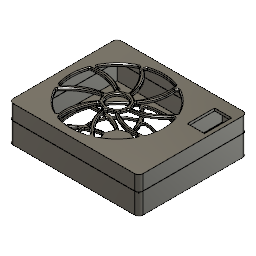
120mm_Solder_Fume_Extractor (Autodesk Fusion 360 design; units mm, degrees)
Autodesk Fusion 360 part; units mm, degrees
sketch "Skizze1" plane through (0, 0, 0) normal (0, 1, 0) x (1, 0, 0)
  circle A0 centre (-52.5, 52.5) radius 2.5
  line L0 (1.75, 0) -> (22.5, 0)
  line L1 (0, -1.75) -> (0, -22.5)
  circle A1 centre (-52.5, -52.5) radius 2.5
  circle A2 centre (52.5, 52.5) radius 2.5
  circle A3 centre (52.5, -52.5) radius 2.5
  line L2 (65, 65) -> (-65, 65)
  line L3 (-65, 65) -> (-65, -65)
  line L4 (-65, -65) -> (65, -65)
  line L5 (65, -65) -> (65, 65)
  line L6 (65, 65) -> (-65, -65) construction
  line L7 (-65, 65) -> (65, -65) construction
  circle A4 centre (0, 0) radius 55
  dimension "d1" = 5
  dimension "d2" = 5
  dimension "d3" = 5
  dimension "d4" = 5
  dimension "d5" = 105
  dimension "d6" = 105
  dimension "d7" = 130
  dimension "d8" = 130
  dimension "d9" = 110
  constraint symmetric A0 L1 A2
  constraint symmetric A0 L0 A1
  constraint symmetric L0 A2 A3
  constraint symmetric L1 A1 A3
  constraint perpendicular L2 L3
  constraint parallel L2 L4
  constraint parallel L3 L5
  constraint horizontal L2
  constraint coincident L6 A4.centre
  constraint coincident L7 A4.centre
  constraint coincident A4.centre origin
  measures "d1" diameter of A0
  measures "d2" diameter of A1
  measures "d3" diameter of A2
  measures "d4" diameter of A3
  measures "d5" vertical distance of A0.centre A1.centre
  measures "d6" horizontal distance of A0.centre A2.centre
  measures "d7" distance of L2.end L3.end
  measures "d8" distance of L3.end L4.end
  measures "d9" diameter of A4
extrude "Extrusion1" add sketch "Skizze1" along normal blind 3 makes body 1
sketch "Skizze2" plane through (0, 0, 0) normal (0, 1, 0) x (1, 0, 0)
  circle A0 centre (0, 0) radius 15
  circle A1 centre (0, 0) radius 55
  arc A2 (0, 0) -> (-18.8111, -51.6831) centre (39.1969, -43.5314) ccw
  arc A3 (0, 0) -> (-21.9924, -50.4117) centre (22.9762, -40.0265) ccw
  dimension "d12" = 30
  constraint coincident A0.centre A1.centre
  measures "d12" diameter of A0
extrude "Extrusion2" add sketch "Skizze2" along normal blind 3 separate body contours A0 A2 A3 | A0 A1 A2 A3 picked at (-8.6621, -7.7901) picked at (-19.3508, -31.0789) makes body 2
sketch "Skizze3" plane through (0, 3, 0) normal (0, 1, 0) x (-1, 0, 0)
  circle A0 centre (-52.5, 52.5) radius 2.5
  circle A1 centre (52.5, -52.5) radius 2.5
  circle A2 centre (-52.5, -52.5) radius 2.5
  circle A3 centre (52.5, 52.5) radius 2.5
  line L0 (-65, 65) -> (-65, -65)
  line L1 (-65, -65) -> (65, -65)
  line L2 (65, -65) -> (65, 65)
  line L3 (65, 65) -> (-65, 65)
  line L4 (65, -65) -> (61, -65)
  line L5 (61, -65) -> (61, 65)
  line L6 (61, 65) -> (65, 65)
  line L7 (65, 65) -> (65, -65)
  line L8 (65, 65) -> (-65, 65)
  line L9 (-65, 65) -> (-65, 61)
  line L10 (-65, 61) -> (65, 61)
  line L11 (65, 61) -> (65, 65)
  line L12 (-65, 65) -> (-61, 65)
  line L13 (-61, 65) -> (-61, -65)
  line L14 (-61, -65) -> (-65, -65)
  line L15 (-65, -65) -> (-65, 65)
  line L16 (-65, -65) -> (65, -65)
  line L17 (65, -65) -> (65, -61)
  line L18 (65, -61) -> (-65, -61)
  line L19 (-65, -61) -> (-65, -65)
  circle A4 centre (0, 0) radius 55
  dimension "d15" = 4
  dimension "d16" = 4
  dimension "d17" = 4
  dimension "d18" = 4
  constraint horizontal L4
  constraint vertical L5
  constraint horizontal L6
  constraint vertical L7
  constraint coincident L1.end L2.start
  constraint horizontal L8
  constraint vertical L9
  constraint horizontal L10
  constraint vertical L11
  constraint horizontal L12
  constraint vertical L13
  constraint horizontal L14
  constraint vertical L15
  constraint horizontal L16
  constraint vertical L17
  constraint horizontal L18
  constraint vertical L19
  constraint coincident L2 L17.end
  measures "d15" distance of L1.end L4.end
  measures "d16" distance of L2.end L10.end
  measures "d17" distance of L0.start L12.end
  measures "d18" distance of L0.end L18.end
extrude "Extrusion3" add sketch "Skizze3" along normal blind 20 contours L0 L3 L8 L9 L10 L12 L13 L15 | L0 L10 L13 L15 L18 | L3 L5 L8 L10 L13 | L0 L1 L13 L14 L15 L16 L18 L19 | L2 L3 L5 L6 L7 L8 L10 L11 | L1 L5 L13 L16 L18 | L2 L5 L7 L10 L18 | L1 L2 L4 L5 L7 L16 L17 L18 bodies 1
sketch "Skizze4" plane through (0, 0, 0) normal (0, 1, 0) x (1, 0, 0)
  line L0 (65, -65) -> (91, -65)
  line L1 (91, -65) -> (91, 65)
  line L2 (91, 65) -> (65, 65)
  line L3 (65, 65) -> (65, -65)
  point P0 (65, -65)
  dimension "d21" = 26
  constraint horizontal L0
  constraint vertical L1
  constraint horizontal L2
  constraint vertical L3
  constraint coincident P0 L0.start
  measures "d21" distance of P0 L0.end
extrude "Extrusion4" add sketch "Skizze4" along normal blind 3 bodies 1
sketch "Skizze5" plane through (0, 3, 0) normal (0, 1, 0) x (-1, 0, 0)
  line L0 (-65, -65) -> (-65, 65)
  line L1 (-65, 65) -> (-91, 65)
  line L2 (-91, 65) -> (-91, -65)
  line L3 (-91, -65) -> (-65, -65)
  line L4 (-91, -65) -> (-65, -65)
  line L5 (-65, -65) -> (-65, -61)
  line L6 (-65, -61) -> (-91, -61)
  line L7 (-91, -61) -> (-91, -65)
  line L8 (-91, 65) -> (-87, 65)
  line L9 (-87, 65) -> (-87, -65)
  line L10 (-87, -65) -> (-91, -65)
  line L11 (-91, -65) -> (-91, 65)
  line L12 (-91, 65) -> (-65, 65)
  line L13 (-65, 65) -> (-65, 61)
  line L14 (-65, 61) -> (-91, 61)
  line L15 (-91, 61) -> (-91, 65)
  dimension "d24" = 4
  dimension "d25" = 4
  dimension "d26" = 4
  constraint horizontal L4
  constraint vertical L5
  constraint horizontal L6
  constraint vertical L7
  constraint coincident L2.end L3.start
  constraint horizontal L8
  constraint vertical L9
  constraint horizontal L10
  constraint vertical L11
  constraint coincident L1.end L2.start
  constraint horizontal L12
  constraint vertical L13
  constraint horizontal L14
  constraint vertical L15
  measures "d24" distance of L2.end L6.end
  measures "d25" distance of L1.end L8.end
  measures "d26" distance of L1.end L14.end
extrude "Extrusion5" add sketch "Skizze5" along normal blind 20 contours L0 L3 L4 L5 L6 L9 | L2 L3 L4 L6 L7 L9 L10 L11 | L0 L1 L9 L12 L13 L14 | L2 L6 L9 L11 L14 | L1 L2 L8 L9 L11 L12 L14 L15 bodies 1
sketch "Skizze6" plane through (0, 0, -61) normal (0, 0, 1) x (1, 0, 0)
  line L0 (65, 3) -> (87, 3)
  line L1 (87, 3) -> (87, 23)
  line L2 (87, 23) -> (65, 23)
  line L3 (65, 23) -> (65, 3)
  line L4 (67, 23) -> (85, 23)
  line L5 (85, 23) -> (85, 21)
  line L6 (85, 21) -> (67, 21)
  line L7 (67, 21) -> (67, 23)
  line L8 (71.5, 21) -> (80.5, 21)
  line L9 (80.5, 21) -> (80.5, 17)
  line L10 (80.5, 17) -> (71.5, 17)
  line L11 (71.5, 17) -> (71.5, 21)
  dimension "d29" = 18
  dimension "d31" = 9
  dimension "d32" = 4
  dimension "d33" = 4.5
  constraint horizontal L4
  constraint vertical L5
  constraint horizontal L6
  constraint vertical L7
  constraint coincident L2 L4.start
  constraint horizontal L8
  constraint vertical L9
  constraint horizontal L10
  constraint vertical L11
  constraint coincident L6 L8.start
  measures "d29" distance of L4.start L4.end
  measures "d31" distance of L8.start L8.end
  measures "d32" distance of L8.start L10.end
  measures "d33" distance of L7 L11
extrude "Extrusion6" cut sketch "Skizze6" against normal blind 4 contours L2 L4 L5 L6 L7 L8 | L6 L8 L9 L10 L11 bodies 1
sketch "Skizze7" plane through (0, 23, 0) normal (0, 1, 0) x (-1, 0, 0)
  line L0 (-61, -61) -> (-61, 61)
  line L1 (-61, 61) -> (61, 61)
  line L2 (61, 61) -> (61, -61)
  line L3 (61, -61) -> (-61, -61)
  line L4 (-65, 61) -> (-65, -61)
  line L5 (-67, -65) -> (65, -65)
  line L6 (65, -65) -> (65, 65)
  line L7 (65, 65) -> (-91, 65)
  line L8 (65, 65) -> (63, 65)
  line L9 (63, -65) -> (65, -65)
  line L10 (65, -65) -> (65, 65)
  line L11 (65, 65) -> (-65, 65)
  line L12 (-65, 65) -> (-65, 63.2)
  line L13 (-65, 63.2) -> (65, 63.2)
  line L14 (65, 63.2) -> (65, 65)
  line L15 (65, -65) -> (-65, -65)
  line L16 (-65, -65) -> (-65, -63)
  line L17 (65, -63) -> (65, -65)
  line L18 (65, 65) -> (63.2, 65)
  line L19 (63.2, 65) -> (63.2, -65)
  line L20 (63.2, -65) -> (65, -65)
  line L21 (65, -65) -> (65, 65)
  line L22 (65, -65) -> (-65, -65)
  line L23 (-65, -65) -> (-65, -63.2)
  line L24 (-65, -63.2) -> (65, -63.2)
  line L25 (65, -63.2) -> (65, -65)
  line L26 (-67, -61) -> (-67, -65)
  line L27 (-91, 65) -> (-91, -65)
  line L28 (-91, -65) -> (-85, -65)
  line L29 (-85, -65) -> (-85, -61)
  line L30 (-85, -61) -> (-87, -61)
  line L31 (-87, -61) -> (-87, 61)
  line L32 (-87, 61) -> (-65, 61)
  line L33 (-65, -61) -> (-67, -61)
  dimension "d36" = 2
  dimension "d37" = 1.8
  dimension "d46" = 1.8
  dimension "d47" = 1.8
  constraint horizontal L8
  constraint horizontal L9
  constraint vertical L10
  constraint coincident L6.end L7.start
  constraint horizontal L11
  constraint vertical L12
  constraint horizontal L13
  constraint vertical L14
  constraint horizontal L15
  constraint vertical L16
  constraint coincident L5.end L6.start
  constraint horizontal L18
  constraint vertical L19
  constraint horizontal L20
  constraint vertical L21
  constraint horizontal L22
  constraint vertical L23
  constraint horizontal L24
  constraint vertical L25
  measures "d36" distance of L6.end L8.end
  measures "d37" distance of L6.end L13.end
  measures "d46" distance of L6.end L18.end
  measures "d47" distance of L5.end L24.end
extrude "Extrusion7" add sketch "Skizze7" along normal blind 2 contours L5 L9 L15 L16 L19 L22 L23 L24 | L5 L6 L9 L10 L15 L17 L19 L20 L21 L22 L24 L25 | L6 L10 L13 L17 L19 L21 L24 | L6 L7 L8 L10 L11 L13 L14 L18 L19 L21 | L7 L8 L11 L12 L13 L19 bodies 1
sketch "Skizze8" plane through (0, 23, 0) normal (0, 1, 0) x (-1, 0, 0)
  line L0 (-85, -65) -> (-85, -61)
  line L1 (-85, -61) -> (-87, -61)
  line L2 (-87, -61) -> (-87, 61)
  line L3 (-87, 61) -> (-65, 61)
  line L4 (-65, 65) -> (-91, 65)
  line L5 (-91, 65) -> (-91, -65)
  line L6 (-91, -65) -> (-85, -65)
  line L7 (-85, -65) -> (-91, -65)
  line L8 (-91, -65) -> (-91, -63.2)
  line L9 (-91, -63.2) -> (-85, -63.2)
  line L10 (-85, -63.2) -> (-85, -65)
  line L11 (-91, -65) -> (-89.2, -65)
  line L12 (-89.2, -65) -> (-89.2, 65)
  line L13 (-89.2, 65) -> (-91, 65)
  line L14 (-91, 65) -> (-91, -65)
  line L15 (-91, 65) -> (-65, 65)
  line L16 (-65, 65) -> (-65, 63.2)
  line L17 (-65, 63.2) -> (-91, 63.2)
  line L18 (-91, 63.2) -> (-91, 65)
  line L19 (-65, -65) -> (-67, -65)
  line L20 (-67, -65) -> (-67, -63.2)
  line L21 (-67, -63.2) -> (-65, -63.2)
  line L22 (-65, -63.2) -> (-65, -65)
  line L23 (-61, -61) -> (-61, 61)
  line L24 (-61, 61) -> (61, 61)
  line L25 (61, 61) -> (61, -61)
  line L26 (61, -61) -> (-61, -61)
  line L27 (-65, -65) -> (-65, -63.2)
  line L28 (-65, -63.2) -> (63.2, -63.2)
  line L29 (63.2, -63.2) -> (63.2, 63.2)
  line L30 (63.2, 63.2) -> (-65, 63.2)
  line L31 (-65, 63.2) -> (-65, 65)
  line L32 (-65, 61) -> (-65, -61)
  line L33 (-65, -61) -> (-67, -61)
  line L34 (-67, -61) -> (-67, -65)
  line L35 (-67, -65) -> (-65, -65)
  point P0 (-91, -65)
  point P1 (-67, -65)
  point P2 (-85, -65)
  point P3 (-65, -65)
  dimension "d40" = 1.8
  dimension "d41" = 1.8
  dimension "d42" = 1.8
  dimension "d43" = 1.8
  constraint horizontal L7
  constraint vertical L8
  constraint horizontal L9
  constraint vertical L10
  constraint coincident P2 L0.start
  constraint horizontal L11
  constraint vertical L12
  constraint horizontal L13
  constraint vertical L14
  constraint coincident P0 L5.end
  constraint horizontal L15
  constraint vertical L16
  constraint horizontal L17
  constraint vertical L18
  constraint horizontal L19
  constraint vertical L20
  constraint horizontal L21
  constraint vertical L22
  measures "d40" distance of P2 L9.end
  measures "d41" distance of P0 L11.end
  measures "d42" distance of L4.end L17.end
  measures "d43" distance of P3 L21.end
extrude "Extrusion8" add sketch "Skizze8" along normal blind 2 contours L0 L6 L7 L9 L10 L12 | L5 L6 L7 L8 L9 L11 L12 L14 | L5 L9 L12 L14 L17 | L4 L5 L12 L13 L14 L15 L17 L18 | L4 L12 L15 L16 L17 L31 | L19 L20 L21 L22 L27 L34 L35 bodies 1
ref_plane "Arbeitsebene2" through (13, 25.2, 0) normal (0, 1, 0) x (0, 0, 1)
sketch "Skizze29" plane through (13, 25.2, 0) normal (0, 1, 0) x (1, 0, 0)
  line L0 (-78, -65) -> (78, -65)
  line L1 (78, -65) -> (78, 65)
  line L2 (78, 65) -> (72, 65)
  line L3 (72, 65) -> (72, 63.2)
  line L4 (72, 63.2) -> (76.2, 63.2)
  line L5 (76.2, 63.2) -> (76.2, -63.2)
  line L6 (76.2, -63.2) -> (-76.2, -63.2)
  line L7 (-76.2, -63.2) -> (-76.2, 63.2)
  line L8 (-76.2, 63.2) -> (54, 63.2)
  line L9 (54, 63.2) -> (54, 65)
  line L10 (54, 65) -> (-78, 65)
  line L11 (-78, 65) -> (-78, -65)
  line L12 (76.2, 63.2) -> (72, 63.2)
  line L13 (72, 63.2) -> (72, 61)
  line L14 (72, 61) -> (74, 61)
  line L15 (74, 61) -> (74, -61)
  line L16 (74, -61) -> (52, -61)
  line L17 (52, -61) -> (52, 61)
  line L18 (52, 61) -> (54, 61)
  line L19 (54, 61) -> (54, 63.2)
  line L20 (54, 63.2) -> (-76.2, 63.2)
  line L21 (-76.2, 63.2) -> (-76.2, -63.2)
  line L22 (-76.2, -63.2) -> (76.2, -63.2)
  line L23 (76.2, -63.2) -> (76.2, 63.2)
  line L24 (48, 61) -> (48, -61)
  line L25 (48, -61) -> (-74, -61)
  line L26 (-74, -61) -> (-74, 61)
  line L27 (-74, 61) -> (48, 61)
  line L28 (54, 61) -> (58.5, 61)
  line L29 (58.5, 61) -> (58.5, 65)
  line L30 (58.5, 65) -> (54, 65)
  line L31 (54, 65) -> (54, 61)
  line L32 (58.5, 61) -> (67.5, 61)
  line L33 (67.5, 61) -> (67.5, 65)
  line L34 (67.5, 65) -> (58.5, 65)
  line L35 (58.5, 65) -> (58.5, 61)
  line L36 (67.5, 61) -> (72, 61)
  line L37 (72, 61) -> (72, 65)
  line L38 (72, 65) -> (67.5, 65)
  line L39 (67.5, 65) -> (67.5, 61)
extrude "Extrusion28" add sketch "Skizze29" along normal blind 15 separate body contours L0 L1 L2 L3 L4 L5 L6 L7 L8 L9 L10 L11 L12 L20 L21 L22 L23 L31 L37 | L9 L19 L28 L29 L30 L31 L35 | L3 L13 L33 L36 L37 L38 L39 | L4 L5 L6 L7 L8 L12 L13 L14 L15 L16 L17 L18 L19 L20 L21 L22 L23 L31 L37 | L29 L32 L33 L34 L35 L39 makes body 3
sketch "Skizze30" plane through (0, 40.2, 0) normal (0, 1, 0) x (-1, 0, 0)
  line L0 (-65, -61) -> (-87, -61)
  line L1 (-87, -61) -> (-87, 61)
  line L2 (-87, 61) -> (-65, 61)
  line L3 (-65, 61) -> (-65, -61)
  line L4 (61, 61) -> (61, -61)
  line L5 (61, -61) -> (-61, -61)
  line L6 (-61, -61) -> (-61, 61)
  line L7 (-61, 61) -> (61, 61)
  line L8 (-91, -65) -> (65, -65)
  line L9 (65, -65) -> (65, 65)
  line L10 (65, 65) -> (-91, 65)
  line L11 (-91, 65) -> (-91, -65)
  line L12 (-87, -61) -> (-65, -61)
  line L13 (-65, -61) -> (-65, 61)
  line L14 (-65, 61) -> (-87, 61)
  line L15 (-87, 61) -> (-87, -61)
  line L16 (61, -61) -> (61, 61)
  line L17 (61, 61) -> (-61, 61)
  line L18 (-61, 61) -> (-61, -61)
  line L19 (-61, -61) -> (61, -61)
  line L20 (65, -65) -> (-91, -65)
  line L21 (-91, -65) -> (-91, 65)
  line L22 (-91, 65) -> (65, 65)
  line L23 (65, 65) -> (65, -65)
  line L24 (-61, -61) -> (61, -61)
  line L25 (61, -61) -> (61, 61)
  line L26 (61, 61) -> (-61, 61)
  line L27 (-61, 61) -> (-61, -61)
  circle A0 centre (-52.5, 52.5) radius 2.5
  circle A1 centre (52.5, -52.5) radius 2.5
  circle A2 centre (-52.5, -52.5) radius 2.5
  circle A3 centre (52.5, 52.5) radius 2.5
  circle A4 centre (0, 0) radius 55
extrude "Extrusion29" add sketch "Skizze30" along normal blind 3 contours L0 L1 L2 L3 L12 L13 L14 L15 | L4 L5 L6 L7 L16 L17 L18 L19 L24 L25 L26 L27 | L8 L9 L10 L11 L20 L21 L22 L23 | A4 bodies 3
sketch "Skizze31" plane through (0, 25.2, 0) normal (0, -1, 0) x (1, 0, 0)
  line L0 (87, -61) -> (65, -61)
  line L1 (65, -61) -> (65, 61)
  line L2 (65, 61) -> (87, 61)
  line L3 (87, 61) -> (87, -61)
  line L4 (-61, -61) -> (-61, 61)
  line L5 (-61, 61) -> (61, 61)
  line L6 (61, 61) -> (61, -61)
  line L7 (61, -61) -> (-61, -61)
  line L8 (-65, -65) -> (91, -65)
  line L9 (91, -65) -> (91, 65)
  line L10 (91, 65) -> (-65, 65)
  line L11 (-65, 65) -> (-65, -65)
  line L12 (-65, 61.0488) -> (91, 61.0488)
  line L13 (91, 61.0488) -> (91, 62.8488)
  line L14 (91, 62.8488) -> (-65, 62.8488)
  line L15 (-65, 62.8488) -> (-65, 61.0488)
  line L16 (87, 62.8488) -> (88.8, 62.8488)
  line L17 (88.8, 62.8488) -> (88.8, -65)
  line L18 (88.8, -65) -> (87, -65)
  line L19 (87, -65) -> (87, 62.8488)
  line L20 (88.8, -61) -> (-65, -61)
  line L21 (-65, -61) -> (-65, -62.8)
  line L22 (-65, -62.8) -> (88.8, -62.8)
  line L23 (88.8, -62.8) -> (88.8, -61)
  line L24 (-61, -62.8) -> (-62.8, -62.8)
  line L25 (-62.8, -62.8) -> (-62.8, 65)
  line L26 (-62.8, 65) -> (-61, 65)
  line L27 (-61, 65) -> (-61, -62.8)
  line L28 (61, 61) -> (65, 61)
  line L29 (65, 61) -> (65, -61)
  line L30 (65, -61) -> (61, -61)
  line L31 (61, -61) -> (61, 61)
  dimension "d160" = 1.8
  dimension "d161" = 1.8
  dimension "d162" = 1.8
  dimension "d163" = 1.8
  constraint horizontal L12
  constraint vertical L13
  constraint horizontal L14
  constraint vertical L15
  constraint coincident L11 L12.start
  constraint horizontal L16
  constraint vertical L17
  constraint horizontal L18
  constraint vertical L19
  constraint coincident L14 L16.start
  constraint horizontal L20
  constraint vertical L21
  constraint horizontal L22
  constraint vertical L23
  constraint coincident L17 L20.start
  constraint horizontal L24
  constraint vertical L25
  constraint horizontal L26
  constraint vertical L27
  constraint coincident L22 L24.start
  constraint horizontal L28
  constraint vertical L29
  constraint horizontal L30
  constraint vertical L31
  constraint coincident L0.end L1.start
  constraint coincident L5.end L6.start
  measures "d160" distance of L12.start L14.end
  measures "d161" distance of L16.start L16.end
  measures "d162" distance of L20.start L22.end
  measures "d163" distance of L24.start L24.end
extrude "Extrusion30" add sketch "Skizze31" along normal blind 2 contours L0 L7 L19 L20 L22 L27 L30 | L17 L19 L20 L22 L23 | L3 L12 L17 L19 L20 | L1 L6 L20 L28 L29 L30 L31 | L12 L14 L16 L17 L19 | L12 L14 L19 L27 | L20 L22 L24 L25 L27 | L4 L12 L20 L25 L27 | L12 L14 L25 L27 bodies 3
sketch "Skizze32" plane through (0, 0, -62.8) normal (0, 0, -1) x (-1, 0, 0)
  line L0 (62.8, 25.2) -> (-88.8, 25.2)
  line L1 (-88.8, 25.2) -> (-88.8, 23.2)
  line L2 (-88.8, 23.2) -> (62.8, 23.2)
  line L3 (62.8, 23.2) -> (62.8, 25.2)
  line L4 (-84.8, 23.2) -> (-67.2274, 23.2)
  line L5 (-67.2274, 23.2) -> (-67.2274, 25.2)
  line L6 (-67.2274, 25.2) -> (-84.8, 25.2)
  line L7 (-84.8, 25.2) -> (-84.8, 23.2)
  line L8 (-67, 25) -> (-67, 21)
  line L9 (-85, 21) -> (-85, 25)
  dimension "d166" = 0.2274
  dimension "d167" = 0.2
  constraint horizontal L4
  constraint vertical L5
  constraint horizontal L6
  constraint vertical L7
  constraint coincident L0 L5.end
  constraint coincident L2 L4.start
  measures "d166" distance of L5 L8
  measures "d167" distance of L7 L9
extrude "Extrusion31" add sketch "Skizze32" along normal blind 2.2 contours L0 L2 L4 L5 L6 L7 bodies 3
extrude "Extrusion32" add 1 faces at (77.5, 17, -63.6667) along direction (0, 1, 0) blind 0.5 on bodies 1 bodies 1
extrude "Extrusion33" add 2 faces at (83.5, 21, -62.3333) (70, 21, -62.3333) along direction (0, 1, 0) blind 0.5 on bodies 1 bodies 1
sketch "Skizze33" plane through (0, 40.2, 0) normal (0, -1, 0) x (1, 0, 0)
  line L0 (65, 61) -> (65, -61)
  line L1 (65, -61) -> (87, -61)
  line L2 (87, -61) -> (87, 61)
  line L3 (87, 61) -> (65, 61)
  line L4 (65.75, -51) -> (86.25, -51)
  line L5 (86.25, -51) -> (86.25, -18.5)
  line L6 (86.25, -18.5) -> (65.75, -18.5)
  line L7 (65.75, -18.5) -> (65.75, -51)
  dimension "d174" = 20.5
  dimension "d175" = 32.5
  dimension "d176" = 0.75
  dimension "d177" = 10
  constraint horizontal L4
  constraint vertical L5
  constraint horizontal L6
  constraint vertical L7
  measures "d174" distance of L4.start L4.end
  measures "d175" distance of L4.start L6.end
  measures "d176" distance of L0 L7
  measures "d177" distance of L1 L4
extrude "Extrusion34" cut sketch "Skizze33" against normal blind 3 contours L4 L5 L6 L7 bodies 3
fillet "Abrundung33" radius 5 8 edges at (91, 12.5, -65) (91, 12.5, 65) (-65, 12.5, 65) (-65, 12.5, -65) (91, 34.2, -65) (91, 34.2, 65) (-65, 34.2, 65) (-65, 34.2, -65) on bodies 1 3
sketch "Skizze35" plane through (0, 43.2, 0) normal (0, 1, 0) x (-1, 0, 0)
  line L0 (-65.75, -51) -> (-86.25, -51)
  line L1 (-86.25, -51) -> (-86.25, -18.5)
  line L2 (-86.25, -18.5) -> (-65.75, -18.5)
  line L3 (-65.75, -18.5) -> (-65.75, -51)
  circle A0 centre (-52.5, 52.5) radius 2.5
  circle A1 centre (52.5, 52.5) radius 2.5
  circle A2 centre (-52.5, -52.5) radius 2.5
  circle A3 centre (52.5, -52.5) radius 2.5
  arc A4 (60, -65) -> (65, -60) centre (60, -60) ccw
  line L4 (65, -60) -> (65, 60)
  arc A5 (65, 60) -> (60, 65) centre (60, 60) ccw
  line L5 (60, 65) -> (-86, 65)
  arc A6 (-86, 65) -> (-91, 60) centre (-86, 60) ccw
  line L6 (-91, 60) -> (-91, -60)
  arc A7 (-91, -60) -> (-86, -65) centre (-86, -60) ccw
  line L7 (-86, -65) -> (60, -65)
  circle A8 centre (52.5, -52.5) radius 2.5
  circle A9 centre (52.5, 52.5) radius 2.5
  circle A10 centre (-52.5, 52.5) radius 2.5
  circle A11 centre (-52.5, -52.5) radius 2.5
extrude "Extrusion36" add sketch "Skizze35" against normal blind 3 contours A0 A10 | A1 A9 | A2 A11 | A3 A8 bodies 3
sketch "Skizze36" plane through (61, 0, 0) normal (-1, 0, 0) x (0, 0, 1)
  line L0 (-61, 3) -> (61, 3)
  line L1 (61, 3) -> (61, 23)
  line L2 (61, 23) -> (-61, 23)
  line L3 (-61, 23) -> (-61, 3)
  circle A0 centre (-35, 9) radius 2
  dimension "d185" = 4
  measures "d185" diameter of A0
extrude "Extrusion37" cut sketch "Skizze36" against normal blind 4 contours A0 bodies 1
sketch "Skizze38" plane through (0, 40.2, 0) normal (0, -1, 0) x (1, 0, 0)
  line L0 (61, 61) -> (-61, 61)
  line L1 (-61, 61) -> (-61, -61)
  line L2 (-61, -61) -> (61, -61)
  line L3 (61, -61) -> (61, 61)
  line L4 (-61, -61) -> (-61, -36)
  line L5 (-61, -61) -> (-36, -61)
  line L6 (-36, -61) -> (-61, -36)
  circle A0 centre (-52.5, -52.5) radius 2.25
  dimension "d194" = 4.5
  constraint coincident L1.end L2.start
  constraint coincident L1 L4.end
  constraint perpendicular L2 L4
  constraint coincident L2 L5.end
  measures "d194" diameter of A0
extrude "Extrusion39" add sketch "Skizze38" along normal blind 8 separate body contours L1 L2 L4 L5 L6 makes body 4
sketch "Skizze39" plane through (0, 40.2, 0) normal (0, 1, 0) x (-1, 0, 0)
  circle A0 centre (52.5, -52.5) radius 2.25
  line L0 (36, -61) -> (61, -61)
  line L1 (61, -61) -> (61, -36)
  line L2 (61, -36) -> (36, -61)
  line L3 (49.5606, -55.4394) -> (53.5759, -56.5153)
  line L4 (53.5759, -56.5153) -> (56.5153, -53.5759)
  line L5 (56.5153, -53.5759) -> (55.4394, -49.5606)
  line L6 (55.4394, -49.5606) -> (51.4241, -48.4847)
  line L7 (51.4241, -48.4847) -> (48.4847, -51.4241)
  line L8 (48.4847, -51.4241) -> (49.5606, -55.4394)
  point P0 (52.5, -52.5)
  dimension "d197" = 7.2
  constraint coincident P0 A0.centre
  measures "d197" distance of L4 L7
extrude "Extrusion40" cut sketch "Skizze39" against normal blind 4 contours L3 L4 L5 L6 L7 L8 bodies 4
copy_body "Körper kopieren/einfügen1" bodies 4 makes body 5
move_body "Verschieben1" bodies 5 to x (0, 0, -1) y (0, 1, 0) z (1, 0, 0) at (0, 0, 0)
copy_body "Körper kopieren/einfügen2" bodies 4 makes body 6
move_body "Verschieben2" bodies 6 to x (-1, 0, 0) y (0, 1, 0) z (0, 0, -1) at (0, 0, 0)
copy_body "Körper kopieren/einfügen3" bodies 4 makes body 7
move_body "Verschieben3" bodies 7 to x (0, 0, 1) y (0, 1, 0) z (-1, 0, 0) at (0, 0, 0)
extrude "Extrusion41" add sketch "Skizze2" along normal blind 3 contours A0 A2 A3 | A0 A1 A2 A3 picked at (-8.6621, -7.7901) picked at (-19.3508, -31.0789) bodies 1
pattern_circular "C-Anordnung1" count 8 over 360 about axis through (0, 1.75, 0) along (0, 1, 0) of bodies 2 makes body 8 at (8.293, 0, 35.6592) makes body 9 at (31.0789, 0, 19.3508) makes body 10 at (35.6592, 0, -8.293) makes body 11 at (19.3508, 0, -31.0789) makes body 12 at (-8.293, 0, -35.6592) makes body 13 at (-31.0789, 0, -19.3508) makes body 14 at (-35.6592, 0, 8.293)
sketch "Skizze40" plane through (0, 0, 0) normal (0, -1, 0) x (1, 0, 0)
  arc A0 (-65, -60) -> (-60, -65) centre (-60, -60) ccw
  line L0 (-60, -65) -> (86, -65)
  arc A1 (86, -65) -> (91, -60) centre (86, -60) ccw
  line L1 (91, -60) -> (91, 60)
  arc A2 (91, 60) -> (86, 65) centre (86, 60) ccw
  line L2 (86, 65) -> (-60, 65)
  arc A3 (-60, 65) -> (-65, 60) centre (-60, 60) ccw
  line L3 (-65, 60) -> (-65, -60)
  circle A4 centre (52.5, 52.5) radius 2.5
  arc A5 (-21.9924, 50.4117) -> (-18.8111, 51.6831) centre (0, 0) ccw
  arc A6 (-21.9924, 50.4117) -> (0, 0) centre (22.9762, 40.0265) ccw
  arc A7 (-18.8111, 51.6831) -> (0, 0) centre (39.1969, 43.5314) ccw
  circle A8 centre (-52.5, -52.5) radius 2.5
  circle A9 centre (52.5, -52.5) radius 2.5
  circle A10 centre (-52.5, 52.5) radius 2.5
  circle A11 centre (0, 0) radius 15
  dimension "d207" = 30
  constraint concentric A5 A11
  measures "d207" diameter of A11
extrude "Extrusion42" add sketch "Skizze40" against normal blind 3 contours A6 A7 A11 picked at (0.895, 5.7134) bodies 8 1 2 9 10 11 12 13 14
fillet "Abrundung34" radius 2 16 edges at (23.244, 1.5, 49.8469) (20.0955, 1.5, 51.1974) (50.4117, 1.5, 21.9924) (51.6831, 1.5, 18.8111) (49.8469, 1.5, -23.244) (51.1974, 1.5, -20.0955) (21.9924, 1.5, -50.4117) (-20.0955, 1.5, -51.1974) (18.8111, 1.5, -51.6831) (-23.244, 1.5, -49.8469) (-50.4117, 1.5, -21.9924) (-51.1974, 1.5, 20.0955) (-21.9924, 1.5, 50.4117) (-49.8469, 1.5, 23.244) (-51.6831, 1.5, -18.8111) (-18.8111, 1.5, 51.6831) on bodies 8
fillet "Abrundung35" radius 2 15 edges at (-14.9567, 1.5, 1.1395) (-11.3817, 1.5, -9.7702) (-11.6226, 1.5, 9.4823) (-1.5134, 1.5, 14.9235) (-9.7702, 1.5, 11.3817) (1.1395, 1.5, 14.9567) (9.4823, 1.5, 11.6226) (11.3817, 1.5, 9.7702) (14.9235, 1.5, 1.5134) (11.6226, 1.5, -9.4823) (1.5134, 1.5, -14.9235) (14.9567, 1.5, -1.1395) (-9.4823, 1.5, -11.6226) (-1.1395, 1.5, -14.9567) (-14.9235, 1.5, -1.5134) on bodies 8
sketch "Skizze41" plane through (0, 43.2, 0) normal (0, 1, 0) x (-1, 0, 0)
  line L0 (-65.75, -51) -> (-86.25, -51)
  line L1 (-86.25, -51) -> (-86.25, -18.5)
  line L2 (-86.25, -18.5) -> (-65.75, -18.5)
  line L3 (-65.75, -18.5) -> (-65.75, -51)
  arc A0 (60, -65) -> (65, -60) centre (60, -60) ccw
  line L4 (65, -60) -> (65, 60)
  arc A1 (65, 60) -> (60, 65) centre (60, 60) ccw
  line L5 (60, 65) -> (-86, 65)
  arc A2 (-86, 65) -> (-91, 60) centre (-86, 60) ccw
  line L6 (-91, 60) -> (-91, -60)
  arc A3 (-91, -60) -> (-86, -65) centre (-86, -60) ccw
  line L7 (-86, -65) -> (60, -65)
  arc A4 (14.6659, 3.1481) -> (12.5047, 8.2845) centre (0, 0) ccw
  arc A5 (14.6659, 3.1481) -> (17.1006, 1.6261) centre (16.6214, 3.5679) ccw
  arc A6 (17.1006, 1.6261) -> (49.082, 22.2512) centre (3.0649, 58.4978) ccw
  arc A7 (49.082, 22.2512) -> (49.3037, 24.3751) centre (47.5108, 23.4887) ccw
  arc A8 (49.3037, 24.3751) -> (25.6141, 48.6716) centre (0, 0) ccw
  arc A9 (25.6141, 48.6716) -> (22.7031, 46.6161) centre (24.6826, 46.9017) ccw
  arc A10 (12.629, 10.6616) -> (22.7031, 46.6161) centre (-22.9762, 40.0265) ccw
  arc A11 (12.629, 10.6616) -> (12.5047, 8.2845) centre (14.172, 9.3891) ccw
  arc A12 (12.5964, -8.1443) -> (14.7002, -2.9841) centre (0, 0) ccw
  arc A13 (12.5964, -8.1443) -> (13.2418, -10.9421) centre (14.276, -9.2302) ccw
  arc A14 (13.2418, -10.9421) -> (50.4402, -18.9722) centre (43.5314, 39.1969) ccw
  arc A15 (50.4402, -18.9722) -> (52.0988, -17.6272) centre (50.2043, -16.9862) ccw
  arc A16 (52.0988, -17.6272) -> (52.5279, 16.3041) centre (0, 0) ccw
  arc A17 (52.5279, 16.3041) -> (49.0161, 16.909) centre (50.6178, 15.7112) ccw
  arc A18 (16.469, -1.3911) -> (49.0161, 16.909) centre (12.0563, 44.5497) ccw
  arc A19 (16.469, -1.3911) -> (14.7002, -2.9841) centre (16.6602, -3.382) ccw
  arc A20 (-3.1481, 14.6659) -> (-8.2845, 12.5047) centre (0, 0) ccw
  arc A21 (-3.1481, 14.6659) -> (-1.6261, 17.1006) centre (-3.5679, 16.6214) ccw
  arc A22 (-1.6261, 17.1006) -> (-22.2512, 49.082) centre (-58.4978, 3.0649) ccw
  arc A23 (-22.2512, 49.082) -> (-24.3751, 49.3037) centre (-23.4887, 47.5108) ccw
  arc A24 (-24.3751, 49.3037) -> (-48.6716, 25.6141) centre (0, 0) ccw
  arc A25 (-48.6716, 25.6141) -> (-46.6161, 22.7031) centre (-46.9017, 24.6826) ccw
  arc A26 (-10.6616, 12.629) -> (-46.6161, 22.7031) centre (-40.0265, -22.9762) ccw
  arc A27 (-10.6616, 12.629) -> (-8.2845, 12.5047) centre (-9.3891, 14.172) ccw
  arc A28 (-12.5964, 8.1443) -> (-14.7002, 2.9841) centre (0, 0) ccw
  arc A29 (-12.5964, 8.1443) -> (-13.2418, 10.9421) centre (-14.276, 9.2302) ccw
  arc A30 (-13.2418, 10.9421) -> (-50.4402, 18.9722) centre (-43.5314, -39.1969) ccw
  arc A31 (-50.4402, 18.9722) -> (-52.0988, 17.6272) centre (-50.2043, 16.9862) ccw
  arc A32 (-52.0988, 17.6272) -> (-52.5279, -16.3041) centre (0, 0) ccw
  arc A33 (-52.5279, -16.3041) -> (-49.0161, -16.909) centre (-50.6178, -15.7112) ccw
  arc A34 (-16.469, 1.3911) -> (-49.0161, -16.909) centre (-12.0563, -44.5497) ccw
  arc A35 (-16.469, 1.3911) -> (-14.7002, 2.9841) centre (-16.6602, 3.382) ccw
  arc A36 (1.3911, 16.469) -> (2.9841, 14.7002) centre (3.382, 16.6602) ccw
  arc A37 (8.1443, 12.5964) -> (2.9841, 14.7002) centre (0, 0) ccw
  arc A38 (8.1443, 12.5964) -> (10.9421, 13.2418) centre (9.2302, 14.276) ccw
  arc A39 (10.9421, 13.2418) -> (18.9722, 50.4402) centre (-39.1969, 43.5314) ccw
  arc A40 (18.9722, 50.4402) -> (17.6272, 52.0988) centre (16.9862, 50.2043) ccw
  arc A41 (17.6272, 52.0988) -> (-16.3041, 52.5279) centre (0, 0) ccw
  arc A42 (-16.3041, 52.5279) -> (-16.909, 49.0161) centre (-15.7112, 50.6178) ccw
  arc A43 (1.3911, 16.469) -> (-16.909, 49.0161) centre (-44.5497, 12.0563) ccw
  circle A44 centre (52.5, 52.5) radius 2.5
  circle A45 centre (-52.5, -52.5) radius 2.5
  circle A46 centre (52.5, -52.5) radius 2.5
  circle A47 centre (-52.5, 52.5) radius 2.5
  arc A48 (60, -65) -> (65, -60) centre (60, -60) ccw
  line L8 (60, -65) -> (-86, -65)
  arc A49 (-91, -60) -> (-86, -65) centre (-86, -60) ccw
  line L9 (-91, -60) -> (-91, 60)
  arc A50 (-86, 65) -> (-91, 60) centre (-86, 60) ccw
  line L10 (-86, 65) -> (60, 65)
  arc A51 (65, 60) -> (60, 65) centre (60, 60) ccw
  line L11 (65, 60) -> (65, -60)
  arc A52 (-14.6659, -3.1481) -> (-12.5047, -8.2845) centre (0, 0) ccw
  arc A53 (-14.6659, -3.1481) -> (-17.1006, -1.6261) centre (-16.6214, -3.5679) ccw
  arc A54 (-17.1006, -1.6261) -> (-49.082, -22.2512) centre (-3.0649, -58.4978) ccw
  arc A55 (-49.082, -22.2512) -> (-49.3037, -24.3751) centre (-47.5108, -23.4887) ccw
  arc A56 (-49.3037, -24.3751) -> (-25.6141, -48.6716) centre (0, 0) ccw
  arc A57 (-25.6141, -48.6716) -> (-22.7031, -46.6161) centre (-24.6826, -46.9017) ccw
  arc A58 (-12.629, -10.6616) -> (-22.7031, -46.6161) centre (22.9762, -40.0265) ccw
  arc A59 (-12.629, -10.6616) -> (-12.5047, -8.2845) centre (-14.172, -9.3891) ccw
  arc A60 (-9.7702, -11.3817) -> (-2.9841, -14.7002) centre (0, 0) ccw
  arc A61 (-9.7702, -11.3817) -> (-18.9722, -50.4402) centre (39.1969, -43.5314) ccw
  arc A62 (-18.9722, -50.4402) -> (-17.6272, -52.0988) centre (-16.9862, -50.2043) ccw
  arc A63 (-17.6272, -52.0988) -> (16.3041, -52.5279) centre (0, 0) ccw
  arc A64 (16.3041, -52.5279) -> (16.909, -49.0161) centre (15.7112, -50.6178) ccw
  arc A65 (-1.3911, -16.469) -> (16.909, -49.0161) centre (44.5497, -12.0563) ccw
  arc A66 (-1.3911, -16.469) -> (-2.9841, -14.7002) centre (-3.382, -16.6602) ccw
  arc A67 (3.1481, -14.6659) -> (8.2845, -12.5047) centre (0, 0) ccw
  arc A68 (3.1481, -14.6659) -> (1.6261, -17.1006) centre (3.5679, -16.6214) ccw
  arc A69 (1.6261, -17.1006) -> (22.2512, -49.082) centre (58.4978, -3.0649) ccw
  arc A70 (22.2512, -49.082) -> (24.3751, -49.3037) centre (23.4887, -47.5108) ccw
  arc A71 (24.3751, -49.3037) -> (48.6716, -25.6141) centre (0, 0) ccw
  arc A72 (48.6716, -25.6141) -> (46.6161, -22.7031) centre (46.9017, -24.6826) ccw
  arc A73 (10.6616, -12.629) -> (46.6161, -22.7031) centre (40.0265, 22.9762) ccw
  arc A74 (10.6616, -12.629) -> (8.2845, -12.5047) centre (9.3891, -14.172) ccw
extrude "Extrusion43" cut sketch "Skizze41" against normal blind 3 contours A4 A5 A6 A7 A8 A9 A10 A11 | A12 A13 A14 A15 A16 A17 A18 A19 | A20 A21 A22 A23 A24 A25 A26 A27 | A28 A29 A30 A31 A32 A33 A34 A35 | A36 A37 A38 A39 A40 A41 A42 A43 | A52 A53 A54 A55 A56 A57 A58 A59 | A60 A61 A62 A63 A64 A65 A66 | A67 A68 A69 A70 A71 A72 A73 A74 bodies 3
sketch "Skizze42" plane through (0, 43.2, 0) normal (0, 1, 0) x (-1, 0, 0)
  arc A0 (10.9421, 13.2418) -> (18.9722, 50.4402) centre (-39.1969, 43.5314) ccw
  arc A1 (8.1443, 12.5964) -> (10.9421, 13.2418) centre (9.2302, 14.276) ccw
  arc A2 (8.1443, 12.5964) -> (2.9841, 14.7002) centre (0, 0) ccw
  arc A3 (1.3911, 16.469) -> (2.9841, 14.7002) centre (3.382, 16.6602) ccw
  arc A4 (1.3911, 16.469) -> (-16.909, 49.0161) centre (-44.5497, 12.0563) ccw
  arc A5 (-16.3041, 52.5279) -> (-16.909, 49.0161) centre (-15.7112, 50.6178) ccw
  arc A6 (17.6272, 52.0988) -> (-16.3041, 52.5279) centre (0, 0) ccw
  arc A7 (18.9722, 50.4402) -> (17.6272, 52.0988) centre (16.9862, 50.2043) ccw
  arc A8 (-18.9722, -50.4402) -> (-17.6272, -52.0988) centre (-16.9862, -50.2043) ccw
  arc A9 (-9.7702, -11.3817) -> (-18.9722, -50.4402) centre (39.1969, -43.5314) ccw
  arc A10 (-9.7702, -11.3817) -> (-2.9841, -14.7002) centre (0, 0) ccw
  arc A11 (-1.3911, -16.469) -> (-2.9841, -14.7002) centre (-3.382, -16.6602) ccw
  arc A12 (-1.3911, -16.469) -> (16.909, -49.0161) centre (44.5497, -12.0563) ccw
  arc A13 (16.3041, -52.5279) -> (16.909, -49.0161) centre (15.7112, -50.6178) ccw
  arc A14 (-17.6272, -52.0988) -> (16.3041, -52.5279) centre (0, 0) ccw
  arc A15 (-17.1006, -1.6261) -> (-49.082, -22.2512) centre (-3.0649, -58.4978) ccw
  arc A16 (-14.6659, -3.1481) -> (-17.1006, -1.6261) centre (-16.6214, -3.5679) ccw
  arc A17 (-14.6659, -3.1481) -> (-12.5047, -8.2845) centre (0, 0) ccw
  arc A18 (-12.629, -10.6616) -> (-12.5047, -8.2845) centre (-14.172, -9.3891) ccw
  arc A19 (-12.629, -10.6616) -> (-22.7031, -46.6161) centre (22.9762, -40.0265) ccw
  arc A20 (-25.6141, -48.6716) -> (-22.7031, -46.6161) centre (-24.6826, -46.9017) ccw
  arc A21 (-49.3037, -24.3751) -> (-25.6141, -48.6716) centre (0, 0) ccw
  arc A22 (-49.082, -22.2512) -> (-49.3037, -24.3751) centre (-47.5108, -23.4887) ccw
  arc A23 (17.1006, 1.6261) -> (49.082, 22.2512) centre (3.0649, 58.4978) ccw
  arc A24 (14.6659, 3.1481) -> (17.1006, 1.6261) centre (16.6214, 3.5679) ccw
  arc A25 (14.6659, 3.1481) -> (12.5047, 8.2845) centre (0, 0) ccw
  arc A26 (12.629, 10.6616) -> (12.5047, 8.2845) centre (14.172, 9.3891) ccw
  arc A27 (12.629, 10.6616) -> (22.7031, 46.6161) centre (-22.9762, 40.0265) ccw
  arc A28 (25.6141, 48.6716) -> (22.7031, 46.6161) centre (24.6826, 46.9017) ccw
  arc A29 (49.3037, 24.3751) -> (25.6141, 48.6716) centre (0, 0) ccw
  arc A30 (49.082, 22.2512) -> (49.3037, 24.3751) centre (47.5108, 23.4887) ccw
  arc A31 (-1.6261, 17.1006) -> (-22.2512, 49.082) centre (-58.4978, 3.0649) ccw
  arc A32 (-3.1481, 14.6659) -> (-1.6261, 17.1006) centre (-3.5679, 16.6214) ccw
  arc A33 (-3.1481, 14.6659) -> (-8.2845, 12.5047) centre (0, 0) ccw
  arc A34 (-10.6616, 12.629) -> (-8.2845, 12.5047) centre (-9.3891, 14.172) ccw
  arc A35 (-10.6616, 12.629) -> (-46.6161, 22.7031) centre (-40.0265, -22.9762) ccw
  arc A36 (-48.6716, 25.6141) -> (-46.6161, 22.7031) centre (-46.9017, 24.6826) ccw
  arc A37 (-24.3751, 49.3037) -> (-48.6716, 25.6141) centre (0, 0) ccw
  arc A38 (-22.2512, 49.082) -> (-24.3751, 49.3037) centre (-23.4887, 47.5108) ccw
  arc A39 (1.6261, -17.1006) -> (22.2512, -49.082) centre (58.4978, -3.0649) ccw
  arc A40 (3.1481, -14.6659) -> (1.6261, -17.1006) centre (3.5679, -16.6214) ccw
  arc A41 (3.1481, -14.6659) -> (8.2845, -12.5047) centre (0, 0) ccw
  arc A42 (10.6616, -12.629) -> (8.2845, -12.5047) centre (9.3891, -14.172) ccw
  arc A43 (10.6616, -12.629) -> (46.6161, -22.7031) centre (40.0265, 22.9762) ccw
  arc A44 (48.6716, -25.6141) -> (46.6161, -22.7031) centre (46.9017, -24.6826) ccw
  arc A45 (24.3751, -49.3037) -> (48.6716, -25.6141) centre (0, 0) ccw
  arc A46 (22.2512, -49.082) -> (24.3751, -49.3037) centre (23.4887, -47.5108) ccw
  arc A47 (-13.2418, 10.9421) -> (-50.4402, 18.9722) centre (-43.5314, -39.1969) ccw
  arc A48 (-12.5964, 8.1443) -> (-13.2418, 10.9421) centre (-14.276, 9.2302) ccw
  arc A49 (-12.5964, 8.1443) -> (-14.7002, 2.9841) centre (0, 0) ccw
  arc A50 (-16.469, 1.3911) -> (-14.7002, 2.9841) centre (-16.6602, 3.382) ccw
  arc A51 (-16.469, 1.3911) -> (-49.0161, -16.909) centre (-12.0563, -44.5497) ccw
  arc A52 (-52.5279, -16.3041) -> (-49.0161, -16.909) centre (-50.6178, -15.7112) ccw
  arc A53 (-52.0988, 17.6272) -> (-52.5279, -16.3041) centre (0, 0) ccw
  arc A54 (-50.4402, 18.9722) -> (-52.0988, 17.6272) centre (-50.2043, 16.9862) ccw
  arc A55 (13.2418, -10.9421) -> (50.4402, -18.9722) centre (43.5314, 39.1969) ccw
  arc A56 (12.5964, -8.1443) -> (13.2418, -10.9421) centre (14.276, -9.2302) ccw
  arc A57 (12.5964, -8.1443) -> (14.7002, -2.9841) centre (0, 0) ccw
  arc A58 (16.469, -1.3911) -> (14.7002, -2.9841) centre (16.6602, -3.382) ccw
  arc A59 (16.469, -1.3911) -> (49.0161, 16.909) centre (12.0563, 44.5497) ccw
  arc A60 (52.5279, 16.3041) -> (49.0161, 16.909) centre (50.6178, 15.7112) ccw
  arc A61 (52.0988, -17.6272) -> (52.5279, 16.3041) centre (0, 0) ccw
  arc A62 (50.4402, -18.9722) -> (52.0988, -17.6272) centre (50.2043, -16.9862) ccw
  line L0 (-65.75, -51) -> (-86.25, -51)
  line L1 (-86.25, -51) -> (-86.25, -18.5)
  line L2 (-86.25, -18.5) -> (-65.75, -18.5)
  line L3 (-65.75, -18.5) -> (-65.75, -51)
  arc A63 (60, -65) -> (65, -60) centre (60, -60) ccw
  line L4 (65, -60) -> (65, 60)
  arc A64 (65, 60) -> (60, 65) centre (60, 60) ccw
  line L5 (60, 65) -> (-86, 65)
  arc A65 (-86, 65) -> (-91, 60) centre (-86, 60) ccw
  line L6 (-91, 60) -> (-91, -60)
  arc A66 (-91, -60) -> (-86, -65) centre (-86, -60) ccw
  line L7 (-86, -65) -> (60, -65)
  circle A67 centre (0, 0) radius 11
  dimension "d215" = 22
  constraint concentric A2 A67
  measures "d215" diameter of A67
extrude "Extrusion44" cut sketch "Skizze42" against normal blind 3 contours A67 bodies 3
sketch "Skizze43" plane through (0, 0, 0) normal (0, -1, 0) x (1, 0, 0)
  arc A0 (-12.5047, 8.2845) -> (-14.6659, 3.1481) centre (0, 0) ccw
  arc A1 (-17.1006, 1.6261) -> (-14.6659, 3.1481) centre (-16.6214, 3.5679) ccw
  arc A2 (-49.082, 22.2512) -> (-17.1006, 1.6261) centre (-3.0649, 58.4978) ccw
  arc A3 (-49.3037, 24.3751) -> (-49.082, 22.2512) centre (-47.5108, 23.4887) ccw
  arc A4 (-25.6141, 48.6716) -> (-49.3037, 24.3751) centre (0, 0) ccw
  arc A5 (-22.7031, 46.6161) -> (-25.6141, 48.6716) centre (-24.6826, 46.9017) ccw
  arc A6 (-22.7031, 46.6161) -> (-12.629, 10.6616) centre (22.9762, 40.0265) ccw
  arc A7 (-12.5047, 8.2845) -> (-12.629, 10.6616) centre (-14.172, 9.3891) ccw
  arc A8 (-14.7002, -2.9841) -> (-12.5964, -8.1443) centre (0, 0) ccw
  arc A9 (-13.2418, -10.9421) -> (-12.5964, -8.1443) centre (-14.276, -9.2302) ccw
  arc A10 (-50.4402, -18.9722) -> (-13.2418, -10.9421) centre (-43.5314, 39.1969) ccw
  arc A11 (-52.0988, -17.6272) -> (-50.4402, -18.9722) centre (-50.2043, -16.9862) ccw
  arc A12 (-52.5279, 16.3041) -> (-52.0988, -17.6272) centre (0, 0) ccw
  arc A13 (-49.0161, 16.909) -> (-52.5279, 16.3041) centre (-50.6178, 15.7112) ccw
  arc A14 (-49.0161, 16.909) -> (-16.469, -1.3911) centre (-12.0563, 44.5497) ccw
  arc A15 (-14.7002, -2.9841) -> (-16.469, -1.3911) centre (-16.6602, -3.382) ccw
  arc A16 (8.2845, 12.5047) -> (3.1481, 14.6659) centre (0, 0) ccw
  arc A17 (1.6261, 17.1006) -> (3.1481, 14.6659) centre (3.5679, 16.6214) ccw
  arc A18 (22.2512, 49.082) -> (1.6261, 17.1006) centre (58.4978, 3.0649) ccw
  arc A19 (24.3751, 49.3037) -> (22.2512, 49.082) centre (23.4887, 47.5108) ccw
  arc A20 (48.6716, 25.6141) -> (24.3751, 49.3037) centre (0, 0) ccw
  arc A21 (46.6161, 22.7031) -> (48.6716, 25.6141) centre (46.9017, 24.6826) ccw
  arc A22 (46.6161, 22.7031) -> (10.6616, 12.629) centre (40.0265, -22.9762) ccw
  arc A23 (8.2845, 12.5047) -> (10.6616, 12.629) centre (9.3891, 14.172) ccw
  arc A24 (14.7002, 2.9841) -> (12.5964, 8.1443) centre (0, 0) ccw
  arc A25 (13.2418, 10.9421) -> (12.5964, 8.1443) centre (14.276, 9.2302) ccw
  arc A26 (50.4402, 18.9722) -> (13.2418, 10.9421) centre (43.5314, -39.1969) ccw
  arc A27 (52.0988, 17.6272) -> (50.4402, 18.9722) centre (50.2043, 16.9862) ccw
  arc A28 (52.5279, -16.3041) -> (52.0988, 17.6272) centre (0, 0) ccw
  arc A29 (49.0161, -16.909) -> (52.5279, -16.3041) centre (50.6178, -15.7112) ccw
  arc A30 (49.0161, -16.909) -> (16.469, 1.3911) centre (12.0563, -44.5497) ccw
  arc A31 (14.7002, 2.9841) -> (16.469, 1.3911) centre (16.6602, 3.382) ccw
  arc A32 (-2.9841, 14.7002) -> (-1.3911, 16.469) centre (-3.382, 16.6602) ccw
  arc A33 (-2.9841, 14.7002) -> (-8.1443, 12.5964) centre (0, 0) ccw
  arc A34 (-10.9421, 13.2418) -> (-8.1443, 12.5964) centre (-9.2302, 14.276) ccw
  arc A35 (-18.9722, 50.4402) -> (-10.9421, 13.2418) centre (39.1969, 43.5314) ccw
  arc A36 (-17.6272, 52.0988) -> (-18.9722, 50.4402) centre (-16.9862, 50.2043) ccw
  arc A37 (16.3041, 52.5279) -> (-17.6272, 52.0988) centre (0, 0) ccw
  arc A38 (16.909, 49.0161) -> (16.3041, 52.5279) centre (15.7112, 50.6178) ccw
  arc A39 (16.909, 49.0161) -> (-1.3911, 16.469) centre (44.5497, 12.0563) ccw
  circle A40 centre (-52.5, 52.5) radius 2.5
  circle A41 centre (52.5, -52.5) radius 2.5
  circle A42 centre (-52.5, -52.5) radius 2.5
  circle A43 centre (52.5, 52.5) radius 2.5
  arc A44 (-65, -60) -> (-60, -65) centre (-60, -60) ccw
  line L0 (-60, -65) -> (86, -65)
  arc A45 (86, -65) -> (91, -60) centre (86, -60) ccw
  line L1 (91, -60) -> (91, 60)
  arc A46 (91, 60) -> (86, 65) centre (86, 60) ccw
  line L2 (86, 65) -> (-60, 65)
  arc A47 (-60, 65) -> (-65, 60) centre (-60, 60) ccw
  line L3 (-65, 60) -> (-65, -60)
  arc A48 (12.5047, -8.2845) -> (14.6659, -3.1481) centre (0, 0) ccw
  arc A49 (17.1006, -1.6261) -> (14.6659, -3.1481) centre (16.6214, -3.5679) ccw
  arc A50 (49.082, -22.2512) -> (17.1006, -1.6261) centre (3.0649, -58.4978) ccw
  arc A51 (49.3037, -24.3751) -> (49.082, -22.2512) centre (47.5108, -23.4887) ccw
  arc A52 (25.6141, -48.6716) -> (49.3037, -24.3751) centre (0, 0) ccw
  arc A53 (22.7031, -46.6161) -> (25.6141, -48.6716) centre (24.6826, -46.9017) ccw
  arc A54 (22.7031, -46.6161) -> (12.629, -10.6616) centre (-22.9762, -40.0265) ccw
  arc A55 (12.5047, -8.2845) -> (12.629, -10.6616) centre (14.172, -9.3891) ccw
  arc A56 (2.9841, -14.7002) -> (9.7702, -11.3817) centre (0, 0) ccw
  arc A57 (18.9722, -50.4402) -> (9.7702, -11.3817) centre (-39.1969, -43.5314) ccw
  arc A58 (17.6272, -52.0988) -> (18.9722, -50.4402) centre (16.9862, -50.2043) ccw
  arc A59 (-16.3041, -52.5279) -> (17.6272, -52.0988) centre (0, 0) ccw
  arc A60 (-16.909, -49.0161) -> (-16.3041, -52.5279) centre (-15.7112, -50.6178) ccw
  arc A61 (-16.909, -49.0161) -> (1.3911, -16.469) centre (-44.5497, -12.0563) ccw
  arc A62 (2.9841, -14.7002) -> (1.3911, -16.469) centre (3.382, -16.6602) ccw
  arc A63 (-8.2845, -12.5047) -> (-3.1481, -14.6659) centre (0, 0) ccw
  arc A64 (-1.6261, -17.1006) -> (-3.1481, -14.6659) centre (-3.5679, -16.6214) ccw
  arc A65 (-22.2512, -49.082) -> (-1.6261, -17.1006) centre (-58.4978, -3.0649) ccw
  arc A66 (-24.3751, -49.3037) -> (-22.2512, -49.082) centre (-23.4887, -47.5108) ccw
  arc A67 (-48.6716, -25.6141) -> (-24.3751, -49.3037) centre (0, 0) ccw
  arc A68 (-46.6161, -22.7031) -> (-48.6716, -25.6141) centre (-46.9017, -24.6826) ccw
  arc A69 (-46.6161, -22.7031) -> (-10.6616, -12.629) centre (-40.0265, 22.9762) ccw
  arc A70 (-8.2845, -12.5047) -> (-10.6616, -12.629) centre (-9.3891, -14.172) ccw
  circle A71 centre (0, 0) radius 34
  circle A72 centre (0, 0) radius 36
  dimension "d218" = 68
  dimension "d219" = 72
  constraint concentric A0 A71
  constraint concentric A71 A72
  measures "d218" diameter of A71
  measures "d219" diameter of A72
extrude "Extrusion45" add sketch "Skizze43" against normal blind 3 contours A2 A6 A71 A72 | A35 A39 A71 A72 | A10 A14 A71 A72 | A18 A22 A71 A72 | A65 A69 A71 A72 | A26 A30 A71 A72 | A57 A61 A71 A72 | A50 A54 A71 A72 bodies 8
fillet "Abrundung36" radius 2 31 edges at (-3.8316, 1.5, -33.7834) (21.7594, 1.5, -28.6797) (-4.8934, 1.5, -35.6659) (17.5767, 1.5, -29.1043) (33.0084, 1.5, -8.1513) (34.7901, 1.5, -9.2546) (18.0564, 1.5, -31.1443) (-9.2546, 1.5, -34.7901) (21.1791, 1.5, -26.5978) (29.1043, 1.5, 17.5767) (-21.1791, 1.5, 26.5978) (-35.6659, 1.5, 4.8934) (-28.6797, 1.5, -21.7594) (33.7834, 1.5, -3.8316) (4.8934, 1.5, 35.6659) (-29.1043, 1.5, -17.5767) (-34.7901, 1.5, 9.2546) (-31.1443, 1.5, -18.0564) (-21.7594, 1.5, 28.6797) (26.5978, 1.5, 21.1791) (28.6797, 1.5, 21.7594) (35.6659, 1.5, -4.8934) (31.1443, 1.5, 18.0564) (9.2546, 1.5, 34.7901) (8.1513, 1.5, 33.0084) (-33.0084, 1.5, 8.1513) (-17.5767, 1.5, 29.1043) (-18.0564, 1.5, 31.1443) (3.8316, 1.5, 33.7834) (-26.5978, 1.5, -21.1791) (-33.7834, 1.5, 3.8316) on bodies 8
chamfer "Fase3" distance 1 angle 45 126 edges at (29.5037, 3, -20.6284) (35.3013, 3, -10.5242) (43.4839, 3, -16.0986) (49.5, 3, -23.2811) (39.3795, 3, -38.396) (23.529, 3, -48.5354) (23.1409, 3, -38.2277) (22.1121, 3, -28.8063) (42.1312, 3, 19.3643) (51.464, 3, 18.5396) (54.9956, 3, 0.6955) (50.9573, 3, -17.6822) (43.3942, 3, -10.668) (36.0048, 3, -4.7335) (35.4488, 3, 6.2757) (32.4036, 3, 17.52) (38.396, 3, 39.3795) (48.5354, 3, 23.529) (38.2277, 3, 23.1409) (28.8063, 3, 22.1121) (20.6284, 3, 29.5037) (10.5242, 3, 35.3013) (16.0986, 3, 43.4839) (23.2811, 3, 49.5) (20.2073, 3, 14.5373) (28.9123, 3, 17.0885) (33.049, 3, 7.9853) (33.0556, 3, -2.4118) (23.9795, 3, 0.0358) (15.3218, 3, 1.8958) (13.89, 3, 5.6628) (12.3271, 3, 9.6798) (13.8259, 3, -5.8176) (15.5612, 3, -1.872) (24.5682, 3, -4.0093) (32.5275, 3, -8.3607) (29.0156, 3, -17.7227) (21.6684, 3, -25.0792) (16.9814, 3, -16.9307) (12.1747, 3, -9.4936) (14.0902, 3, -19.2031) (17.0885, 3, -28.9123) (7.9853, 3, -33.049) (-2.4118, 3, -33.0556) (0.0358, 3, -23.9795) (1.8958, 3, -15.3218) (6.5895, 3, -13.4751) (-10.668, 3, -43.3942) (-4.7335, 3, -36.0048) (6.2757, 3, -35.4488) (17.52, 3, -32.4036) (19.3643, 3, -42.1312) (18.5396, 3, -51.464) (0.6955, 3, -54.9956) (-17.6822, 3, -50.9573) (-0.6955, 3, 54.9956) (17.6822, 3, 50.9573) (10.668, 3, 43.3942) (4.7335, 3, 36.0048) (-6.2757, 3, 35.4488) (-17.52, 3, 32.4036) (-19.3643, 3, 42.1312) (-18.5396, 3, 51.464) (-7.9853, 3, 33.049) (2.4118, 3, 33.0556) (-0.0358, 3, 23.9795) (-1.8958, 3, 15.3218) (-5.6628, 3, 13.89) (-9.6798, 3, 12.3271) (-14.5373, 3, 20.2073) (-17.0885, 3, 28.9123) (-29.0156, 3, 17.7227) (-21.6684, 3, 25.0792) (-16.9814, 3, 16.9307) (-12.1747, 3, 9.4936) (-13.8259, 3, 5.8176) (-15.5612, 3, 1.872) (-24.5682, 3, 4.0093) (-32.5275, 3, 8.3607) (-39.3795, 3, 38.396) (-23.529, 3, 48.5354) (-23.1409, 3, 38.2277) (-22.1121, 3, 28.8063) (-29.5037, 3, 20.6284) (-35.3013, 3, 10.5242) (-43.4839, 3, 16.0986) (-49.5, 3, 23.2811) (-13.89, 3, -5.6628) (-12.3271, 3, -9.6798) (-20.2073, 3, -14.5373) (-28.9123, 3, -17.0885) (-33.049, 3, -7.9853) (-33.0556, 3, 2.4118) (-23.9795, 3, -0.0358) (-15.3218, 3, -1.8958) (-4.3019, 3, -25.2952) (-1.872, 3, -15.5612) (-5.8176, 3, -13.8259) (-9.4936, 3, -12.1747) (-16.9307, 3, -16.9814) (-25.0792, 3, -21.6684) (-17.0404, 3, -29.4215) (-38.2277, 3, -23.1409) (-28.8063, 3, -22.1121) (-20.6284, 3, -29.5037) (-10.5242, 3, -35.3013) (-16.0986, 3, -43.4839) (-23.2811, 3, -49.5) (-38.396, 3, -39.3795) (-48.5354, 3, -23.529) (-43.3942, 3, 10.668) (-36.0048, 3, 4.7335) (-35.4488, 3, -6.2757) (-32.4036, 3, -17.52) (-42.1312, 3, -19.3643) (-51.464, 3, -18.5396) (-54.9956, 3, -0.6955) (-50.9573, 3, 17.6822) (5.8176, 3, 13.8259) (1.872, 3, 15.5612) (4.0093, 3, 24.5682) (8.3607, 3, 32.5275) (17.7227, 3, 29.0156) (25.0792, 3, 21.6684) (16.9307, 3, 16.9814) (9.4936, 3, 12.1747) on bodies 8
chamfer "Fase4" distance 1 angle 45 64 edges at (-54.9956, 43.2, -0.6955) (-51.464, 43.2, -18.5396) (-31.1707, 43.2, -18.0621) (-12.3271, 43.2, -9.6798) (-13.89, 43.2, -5.6628) (-15.3218, 43.2, -1.8958) (-34.6759, 43.2, 4.3205) (-50.9573, 43.2, 17.6822) (-38.396, 43.2, -39.3795) (-23.2811, 43.2, -49.5) (-9.2692, 43.2, -34.8128) (-1.872, 43.2, -15.5612) (-5.8176, 43.2, -13.8259) (-9.4936, 43.2, -12.1747) (-27.5746, 43.2, -21.4645) (-48.5354, 43.2, -23.529) (6.5895, 43.2, -13.4751) (1.8958, 43.2, -15.3218) (-4.3205, 43.2, -34.6759) (-17.6822, 43.2, -50.9573) (0.6955, 43.2, -54.9956) (18.5396, 43.2, -51.464) (17.8201, 43.2, -30.0984) (39.3795, 43.2, -38.396) (49.5, 43.2, -23.2811) (34.8128, 43.2, -9.2692) (15.5612, 43.2, -1.872) (13.8259, 43.2, -5.8176) (12.1747, 43.2, -9.4936) (21.4645, 43.2, -27.5746) (23.529, 43.2, -48.5354) (54.9956, 43.2, 0.6955) (51.464, 43.2, 18.5396) (31.1707, 43.2, 18.0621) (12.3271, 43.2, 9.6798) (13.89, 43.2, 5.6628) (15.3218, 43.2, 1.8958) (34.6759, 43.2, -4.3205) (50.9573, 43.2, -17.6822) (38.396, 43.2, 39.3795) (23.2811, 43.2, 49.5) (9.2692, 43.2, 34.8128) (1.872, 43.2, 15.5612) (5.8176, 43.2, 13.8259) (9.4936, 43.2, 12.1747) (27.5746, 43.2, 21.4645) (48.5354, 43.2, 23.529) (-5.6628, 43.2, 13.89) (-1.8958, 43.2, 15.3218) (4.3205, 43.2, 34.6759) (17.6822, 43.2, 50.9573) (-0.6955, 43.2, 54.9956) (-18.5396, 43.2, 51.464) (-18.0621, 43.2, 31.1707) (-9.6798, 43.2, 12.3271) (-13.8259, 43.2, 5.8176) (-12.1747, 43.2, 9.4936) (-21.4645, 43.2, 27.5746) (-23.529, 43.2, 48.5354) (-39.3795, 43.2, 38.396) (-49.5, 43.2, 23.2811) (-34.8128, 43.2, 9.2692) (-15.5612, 43.2, 1.872) (10.2556, 43.2, 3.9778) on bodies 3
equation "d15 = d16"
equation "d17 = d16"
equation "d18 = d16"
equation "d33 = d31 / 2"
equation "d37 = d46"
equation "d40 = d43"
equation "d41 = d43"
equation "d42 = d43"
equation "d47 = d46"
named bodies: "Fan_Case_Bottom", "Fan_Case_Top", "Corner1", "Corner2", "Corner3", "Corner4", "Fan_Case_Back"
